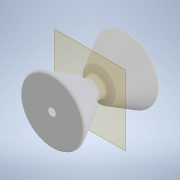
# Autodesk Inventor part: wheel
Saved by Autodesk Inventor 2020 (Build 240168000, 168)
## iProperties
Created: 2022-12-14
Part Number: wheel
Material: Generic
Document SubType Name: Modeling
Designer: Manish
Density: 1 g/cm^3
Appearance: Default
Author: Manish
Autodesk Inventor part; units mm, degrees
ref_plane "YZ Plane" through (0, 0, 0) normal (1, 0, 0) x (0, 1, 0)
ref_plane "XZ Plane" through (0, 0, 0) normal (0, 1, 0) x (-1, 0, 0)
ref_plane "XY Plane" through (0, 0, 0) normal (0, 0, 1) x (1, 0, 0)
sketch "Sketch1" plane through (0, 0, 0) normal (0, 1, 0) x (-1, 0, 0)
  line L0 (0, 0) -> (-31.5359, 0)
  line L1 (0, 0) -> (27.4991, 0) construction
  line L2 (-33.2679, -3) -> (-17.5, -30.3109)
  line L3 (-35, 0) -> (8.6719, 0) construction
  line L4 (0, 0) -> (0, -35)
  arc A0 (-17.5, -30.3109) -> (-11.3514, -33.1081) centre (0, 0) ccw
  line L5 (-10, -35) -> (-10, -45.3109)
  line L6 (0, -45.3109) -> (0, -30.3109)
  line L7 (0, -80) -> (-31.5359, -80)
  line L8 (-33.2679, -77) -> (-17.5, -49.6891)
  line L9 (-35, -80) -> (8.6719, -80) construction
  line L10 (0, -80) -> (0, -45)
  arc A1 (-11.3514, -46.8919) -> (-17.5, -49.6891) centre (0, -80) ccw
  line L11 (-10.0944, -45.6071) -> (-10, -45.3109)
  line L12 (0, -45.3109) -> (0, -49.6891)
  arc A2 (-31.5359, 0) -> (-33.2679, -3) centre (-31.5359, -2) ccw
  arc A3 (-33.2679, -77) -> (-31.5359, -80) centre (-31.5359, -78) ccw
  arc A4 (-10, -35) -> (-11.3514, -33.1081) centre (-12, -35) ccw
  arc A5 (-11.3514, -46.8919) -> (-10.0944, -45.6071) centre (-12, -45) ccw
  line L13 (-4, 0) -> (-4, -80)
  dimension "d0" = 35
  dimension "d3" = 60
  dimension "d5" = 10
  dimension "d7" = 2
  dimension "d8" = 80
  constraints: 28 end point, 14 point on circle, 8 point on line, 8 tangent, 6 centre point, 4 coincident, 3 equal radius, 3 horizontal, 1 parallel, 1 perpendicular, 1 vertical
  measures "d0" distance of L0.start L3.start
  measures "d3" angle of L2 L3
  measures "d5" distance of L6.start L5.end
  measures "d7" radius of A2
  measures "d8" distance between parallel lines of L7 L0
revolve "Revolution1" add sketch "Sketch1" angle 360 about axis through (0, 0, 0) along (0, 0, -1) contours L13 L7 A3 L8 A1 A5 L11 L5 A4 A0 L2 A2 L0
ref_plane "Work Plane1" through (0, 0, -40) normal (0, 0, 1) x (1, 0, 0)
body "Solid1"
